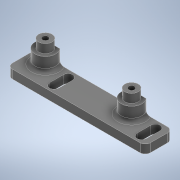
# Autodesk Inventor part: Rack support
Saved by Autodesk Inventor 2022 (Build 260153000, 153)
## iProperties
Created: 2022-03-06
Part Number: Rack support
Material: Genérico
Document SubType Name: Modeling
Designer: JK
Density: 1 g/cm^3
Appearance: Suave - Negro
Author: JK
Autodesk Inventor part; units mm, degrees
ref_plane "YZ Plane" through (0, 0, 0) normal (1, 0, 0) x (0, 1, 0)
ref_plane "XZ Plane" through (0, 0, 0) normal (0, 1, 0) x (-1, 0, 0)
ref_plane "XY Plane" through (0, 0, 0) normal (0, 0, 1) x (1, 0, 0)
sketch "Boceto1" plane through (0, 0, 0) normal (0, 1, 0) x (-1, 0, 0)
  line L0 (-40, 8) -> (40, 8)
  line L1 (40, 8) -> (40, -8)
  line L2 (40, -8) -> (-40, -8)
  line L3 (-40, -8) -> (-40, 8)
  line L4 (-40, 8) -> (40, -8) construction
  line L5 (40, 8) -> (-40, -8) construction
  circle A0 centre (-34, 4) radius 2.7
  circle A1 centre (-34, -4) radius 2.7
  circle A2 centre (16.7, 4) radius 2.7
  circle A3 centre (16.7, -4) radius 2.7
  line L6 (19.4, 4) -> (14, 4)
  line L7 (14, 4) -> (14, -4)
  line L8 (14, -4) -> (19.4, -4)
  line L9 (19.4, -4) -> (19.4, 4)
  line L10 (-31.3, 4) -> (-36.7, 4)
  line L11 (-36.7, 4) -> (-36.7, -4)
  line L12 (-36.7, -4) -> (-31.3, -4)
  line L13 (-31.3, -4) -> (-31.3, 4)
  point P0 (0, 0)
  point P1 (16.7, -4)
  point P2 (16.7, 4)
  point P3 (-34, -4)
  point P4 (-34, 4)
  point P5 (19.4, -4)
  point P6 (-31.3, -4)
  dimension "d2" = 5.4
  dimension "d0" = 80
  dimension "d1" = 16
  dimension "d3" = 4
  dimension "d4" = 8
  dimension "d5" = 6
  dimension "d6" = 50.7
  constraints: 28 end point, 7 midpoint, 6 parallel, 3 horizontal, 3 perpendicular, 3 vertical, 2 horizontal alignment, 1 centre point, 1 point on line, 1 tangent, 1 vertical alignment, 11 other
  measures "d0" distance of L1.end L2.end
  measures "d1" distance of L0.end L1.end
  measures "d3" vertical distance of point (0, 0) point (-34, 4)
  measures "d4" distance of L10.end L11.end
  measures "d5" distance from line of L3 point (-34, 4)
  measures "d6" distance of point (16.7, 4) point (-34, 4)
extrude "Extrusión1" add sketch "Boceto1" along normal blind 5
sketch "Boceto2" plane through (0, 5, 0) normal (0, 1, 0) x (1, 0, 0)
  circle A0 centre (20, 4.1) radius 3.9
  circle A1 centre (-30, 4.1) radius 3.9
  line L0 (40, 8) -> (-40, 8) projected
  line L1 (40, -8) -> (40, 8) projected
  line L2 (-40, 8) -> (-40, -8) projected
  point P0 (0, 0)
  dimension "d11" = 7.8
  dimension "d12" = 20
  dimension "d13" = 10
  constraints: 2 centre point, 2 tangent, 1 equal radius
  measures "d11" diameter of A1
  measures "d12" distance from line of A0.centre L1
  measures "d13" distance from line of L2 A1.centre
extrude "Extrusión2" add sketch "Boceto2" along normal blind 13
sketch "Boceto3" plane through (0, 5, 0) normal (0, 1, 0) x (1, 0, 0)
  line L0 (31.3, -4) -> (31.3, 4) projected
  arc A0 (36.7, 4) -> (31.3, 4) centre (34, 4) ccw projected
  line L1 (36.7, 4) -> (36.7, -4) projected
  arc A1 (31.3, -4) -> (36.7, -4) centre (34, -4) ccw projected
  line L2 (-19.4, -4) -> (-19.4, 4) projected
  arc A2 (-14, 4) -> (-19.4, 4) centre (-16.7, 4) ccw projected
  line L3 (-14, 4) -> (-14, -4) projected
  arc A3 (-19.4, -4) -> (-14, -4) centre (-16.7, -4) ccw projected
  line L4 (40, 8) -> (20, 8) projected
  circle A4 centre (20, 4.1) radius 3.9 projected
  line L5 (20, 8) -> (-30, 8) projected
  circle A5 centre (-30, 4.1) radius 3.9 projected
  line L6 (-30, 8) -> (-40, 8) projected
  line L7 (-40, 8) -> (-40, -8) projected
  line L8 (-40, -8) -> (40, -8) projected
  line L9 (40, -8) -> (40, 8) projected
  circle A6 centre (-30, 4.1) radius 3.9 projected
  circle A7 centre (-30, 4.1) radius 6
  circle A8 centre (20, 4.1) radius 3.9 projected
  circle A9 centre (20, 4.1) radius 6
  point P0 (0, 0)
  point P1 (15.4404, 8)
  point P2 (24.5596, 8)
  point P3 (-34.5596, 8)
  point P4 (-25.4404, 8)
  dimension "d14" = 12
  dimension "d15" = 12
  constraints: 4 vertical alignment, 2 centre point, 2 coincident
  measures "d14" diameter of A7
  measures "d15" diameter of A9
extrude "Extrusión3" add sketch "Boceto3" along normal blind 8 contours A9 L5 L4 | A7 L6 L5 picked at (25.2424, 3.6235) picked at (-24.7576, 3.6235)
fillet "Empalme1" radius 2 2 edges at (20, 5, 1.9) (-30, 5, 1.9)
sketch "Boceto4" plane through (-30, 18, -4.1) normal (0, 1, 0) x (1, 0, 0)
  circle A0 centre (0, 0) radius 3.9 projected
  circle A1 centre (0, 0) radius 1.7
  circle A2 centre (50, 0) radius 3.9 projected
  circle A3 centre (50, 0) radius 1.7
  point P0 (30, -4.1)
  dimension "d19" = 3.4
  dimension "d20" = 3.4
  constraints: 2 centre point, 2 coincident
  measures "d19" diameter of A1
  measures "d20" diameter of A3
extrude "Extrusión4" cut sketch "Boceto4" against normal through all contours A1 | A3
fillet "Empalme2" radius 3 4 edges at (-40, 2.5, 8) (-40, 2.5, -8) (40, 2.5, 8) (40, 2.5, -8)
sketch "Boceto5" plane through (0, 0, 0) normal (0, -1, 0) x (1, 0, 0)
  circle A0 centre (-30, -4.1) radius 1.7 projected
  circle A1 centre (-30, -4.1) radius 2.875
  circle A2 centre (20, -4.1) radius 1.7 projected
  circle A3 centre (20, -4.1) radius 2.875
  line L0 (-33.3198, -4.1) -> (-31.6599, -1.225)
  line L1 (-31.6599, -1.225) -> (-28.3401, -1.225)
  line L2 (-28.3401, -1.225) -> (-26.6802, -4.1)
  line L3 (-26.6802, -4.1) -> (-28.3401, -6.975)
  line L4 (-28.3401, -6.975) -> (-31.6599, -6.975)
  line L5 (-31.6599, -6.975) -> (-33.3198, -4.1)
  line L6 (16.6802, -4.1) -> (18.3401, -1.225)
  line L7 (18.3401, -1.225) -> (21.6599, -1.225)
  line L8 (21.6599, -1.225) -> (23.3198, -4.1)
  line L9 (23.3198, -4.1) -> (21.6599, -6.975)
  line L10 (21.6599, -6.975) -> (18.3401, -6.975)
  line L11 (18.3401, -6.975) -> (16.6802, -4.1)
  point P0 (0, 0)
  dimension "d24" = 5.75
  constraints: 24 end point, 4 coincident, 2 centre point, 2 tangent, 1 equal radius, 1 horizontal, 1 horizontal alignment, 26 other
  measures "d24" diameter of A1
extrude "Extrusión5" cut sketch "Boceto5" against normal blind 5.5 contours A0 | A1 | A1 L2 L3 | A1 L1 L2 | L3 L4 A1 | A1 L0 L1 | L4 L5 A1 | A1 L5 L0 | A2 | A3 | A3 L8 L9 | A3 L7 L8 | L9 L10 A3 | A3 L6 L7 | L10 L11 A3 | A3 L11 L6
